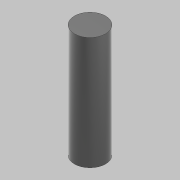
# Autodesk Inventor part: cable
Saved by Autodesk Inventor 2021.4 (Build 254397000, 397)
## iProperties
Created: 2023-05-05
Part Number: cable
Material: PPS-Kunststoff
Document SubType Name: Modeling
Designer: Tilman Preuschoff
Density: 1.637 g/cm^3
Appearance: Glatt - Schwarz
Author: Tilman Preuschoff
Autodesk Inventor part; units mm, degrees
ref_plane "YZ Plane" through (0, 0, 0) normal (1, 0, 0) x (0, 1, 0)
ref_plane "XZ Plane" through (0, 0, 0) normal (0, 1, 0) x (-1, 0, 0)
ref_plane "XY Plane" through (0, 0, 0) normal (0, 0, 1) x (1, 0, 0)
sketch "Skizze1" plane through (0, 0, 0) normal (0, 1, 0) x (-1, 0, 0)
  circle A0 centre (0, 0) radius 2.75
  dimension "d0" = 5.5
  constraints: 1 centre point, 1 coincident
  measures "d0" diameter of A0
extrude "Extrusion1" add sketch "Skizze1" along normal blind 20
